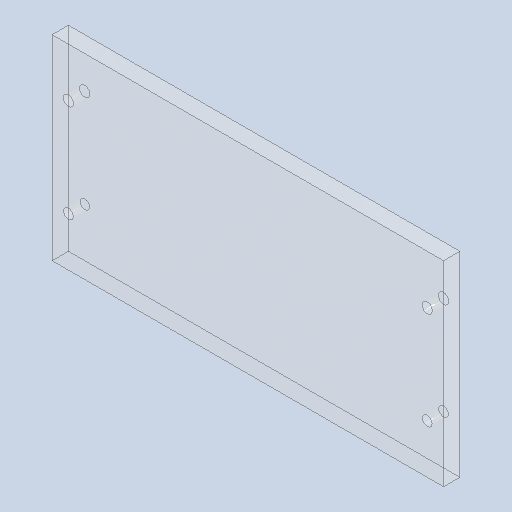
# Autodesk Inventor part: part4
Saved by Autodesk Inventor 2025.2 (Build 292293000, 293)
## iProperties
Created: 2025-02-28
Part Number: part4
Material: アクリル、クリア
Document SubType Name: Modeling
Designer: haruy
Density: 1.19 g/cm^3
Appearance: 透明 - クリア
Author: haruy
Autodesk Inventor part; units mm, degrees
ref_plane "YZ Plane" through (0, 0, 0) normal (1, 0, 0) x (0, 1, 0)
ref_plane "XZ Plane" through (0, 0, 0) normal (0, 1, 0) x (-1, 0, 0)
ref_plane "XY Plane" through (0, 0, 0) normal (0, 0, 1) x (1, 0, 0)
derived "oikon-Sketch-Base.ipt"
sketch "スケッチ2" plane through (0, 0, 0) normal (0, 0, 1) x (1, 0, 0)
  line L0 (0, 0) -> (-100, 0) projected
  line L1 (-100, 0) -> (-100, -50) projected
  line L2 (-100, -50) -> (0, -50) projected
  line L3 (0, -50) -> (0, 0) projected
  line L4 (0, -9) -> (-25.2, -9) projected
  line L5 (-25.2, -9) -> (-25.2, -17) projected
  line L6 (-25.2, -17) -> (0, -17) projected
  line L7 (0, -17) -> (0, -9) projected
  line L8 (0, -50) -> (10, -50) projected
  line L9 (10, -50) -> (10, 0) projected
  line L10 (10, 0) -> (0, 0) projected
  line L11 (0, 0) -> (0, -50) projected
  line L12 (-100, -50) -> (-110, -50) projected
  line L13 (-110, -50) -> (-110, 0) projected
  line L14 (-110, 0) -> (-100, 0) projected
  line L15 (-100, 0) -> (-100, -50) projected
  line L16 (-10.1, -6) -> (-15.1, -6) projected
  line L17 (-15.1, -6) -> (-15.1, -20.9) projected
  line L18 (-15.1, -20.9) -> (-10.1, -20.9) projected
  line L19 (-10.1, -20.9) -> (-10.1, -6) projected
  circle A0 centre (-5, -13) radius 1.6 projected
  line L20 (-12.6, -20.9) -> (-12.6, -6) projected
  circle A1 centre (-20.2, -13) radius 1.6 projected
  line L21 (-37.4, -9) -> (-62.6, -9) projected
  line L22 (-62.6, -9) -> (-62.6, -17) projected
  line L23 (-62.6, -17) -> (-37.4, -17) projected
  line L24 (-37.4, -17) -> (-37.4, -9) projected
  circle A2 centre (-42.4, -13) radius 1.6 projected
  circle A3 centre (-57.6, -13) radius 1.6 projected
  circle A4 centre (-79.8, -13) radius 1.6 projected
  circle A5 centre (-95, -13) radius 1.6 projected
  circle A6 centre (5, -10) radius 1.6 projected
  circle A7 centre (5, -40) radius 1.5 projected
  line L25 (-50, 0) -> (-50, -50) projected
  circle A8 centre (-105, -10) radius 1.6 projected
  circle A9 centre (-105, -40) radius 1.5 projected
  line L26 (-47.5, -6) -> (-52.5, -6) projected
  line L27 (-52.5, -6) -> (-52.5, -40.2) projected
  line L28 (-52.5, -40.2) -> (-47.5, -40.2) projected
  line L29 (-47.5, -40.2) -> (-47.5, -6) projected
  line L30 (-84.9, -6) -> (-89.9, -6) projected
  line L31 (-89.9, -6) -> (-89.9, -35.3712) projected
  line L32 (-89.9, -35.3712) -> (-84.9, -35.3712) projected
  line L33 (-84.9, -35.3712) -> (-84.9, -6) projected
  line L34 (10, 0) -> (-110, 0) projected
  line L35 (-110, 0) -> (-110, 5) projected
  line L36 (-110, 5) -> (10, 5) projected
  line L37 (10, 5) -> (10, 0) projected
  line L38 (10, -50) -> (-110, -50) projected
  line L39 (-110, -50) -> (-110, -55) projected
  line L40 (-110, -55) -> (10, -55) projected
  line L41 (10, -55) -> (10, -50) projected
  circle A10 centre (-5, -5) radius 1.6 projected
  line L42 (10, -25) -> (-100, -25) projected
  circle A11 centre (-5, -45) radius 1.6 projected
  circle A12 centre (-95, -45) radius 1.6 projected
  circle A13 centre (-95, -5) radius 1.6 projected
  line L43 (-15.2, -5.9) -> (-10, -5.9) projected
  line L44 (-10, -5.9) -> (-10, -21) projected
  line L45 (-10, -21) -> (-15.2, -21) projected
  line L46 (-15.2, -21) -> (-15.2, -5.9) projected
  line L47 (-9.6, -40.2) -> (-15.6, -40.2) projected
  line L48 (-15.6, -40.2) -> (-15.6, -21) projected
  line L49 (-15.6, -21) -> (-9.6, -21) projected
  line L50 (-9.6, -21) -> (-9.6, -40.2) projected
  line L51 (-53, -40.2) -> (-53, -21) projected
  line L52 (-47, -40.2) -> (-53, -40.2) projected
  line L53 (-47, -21) -> (-47, -40.2) projected
  line L54 (-53, -21) -> (-47, -21) projected
  line L55 (-47.4, -5.9) -> (-47.4, -21) projected
  line L56 (-52.6, -21) -> (-52.6, -5.9) projected
  line L57 (-52.6, -5.9) -> (-47.4, -5.9) projected
  line L58 (-90.4, -40.2) -> (-90.4, -21) projected
  line L59 (-84.4, -40.2) -> (-90.4, -40.2) projected
  line L60 (-84.4, -21) -> (-84.4, -40.2) projected
  line L61 (-90.4, -21) -> (-84.4, -21) projected
  line L62 (-84.8, -5.9) -> (-84.8, -21) projected
  line L63 (-90, -21) -> (-90, -5.9) projected
  line L64 (-90, -5.9) -> (-84.8, -5.9) projected
  point P0 (-84.9, -21)
  point P1 (-89.9, -21)
  point P2 (-52.5, -9)
  point P3 (-52.6, -9)
  point P4 (-47.4, -9)
  point P5 (-47.5, -9)
  point P6 (-52.5, -17)
  point P7 (-52.6, -17)
  point P8 (-47.5, -17)
  point P9 (-47.4, -17)
  constraints: 2 horizontal
extrude "押し出し1" add sketch "スケッチ2" along normal blind 5 contours L3 L4 L44 L43 L46 L5 L6 L49 L48 L42 L53 L54 L55 L23 L24 L21 L57 L25 L0 | L10 L9 L42 L3 | L0 L14 L35 L36 L37 L10 | L25 L57 L56 L21 L22 L23 L54 L51 L42 L60 L61 L62 L64 L63 L58 L1 L0 | L3 L6 L44 L4 | L1 L12 L13 L14 | L57 L55 L21 L29 L26 L25 | L25 L26 L27 L21 L56 L57 | L3 L42 L50 L49 L44 L6 | L44 L6 L19 L4 | L4 L19 L16 L17 L46 L43 L44 | L9 L8 L3 L42 | L42 L58 L59 L60 L51 L52 L28 L25 L2 L1 | L26 L29 L21 L25 | L25 L21 L27 L26 | L3 L2 L25 L28 L52 L53 L42 L48 L47 L50 | L44 L45 L46 L6 L17 L18 L19 | L19 L6 L20 L4 | L4 L20 L16 L19 | L41 L40 L39 L12 L2 L8 | L58 L61 L31 L42 | L42 L31 L32 L33 L60 L59 L58 | L25 L23 L27 L21 | L21 L29 L23 L25 | L56 L23 L22 L21 | L21 L27 L23 L56 | L55 L23 L29 L21 | L21 L24 L23 L55 | L50 L47 L48 L42 | L42 L48 L49 L45 L50 | L19 L18 L20 L6 | L20 L6 L17 L4 | L4 L17 L16 L20 | L42 L33 L32 L31 | L31 L61 L33 L42 | L25 L54 L27 L23 | L23 L29 L54 L25 | L23 L27 L54 L56 | L55 L54 L29 L23 | L20 L18 L17 L6 | L17 L6 L46 L4 | L46 L6 L5 L4 | L28 L27 L42 L25 | L25 L42 L29 L28 | L61 L63 L64 L62 L33 L30 L31 | L31 L30 L33 L61 | L33 L61 L60 L42 | L54 L29 L42 L25 | L25 L42 L27 L54 | L54 L27 L42 L51 | L54 L53 L42 L29 | L53 L52 L29 L42 | L52 L51 L42 L27 | A0 | A1 | A2 | A3 | A4 | A5 | A10 | A11 | A12 | A13
